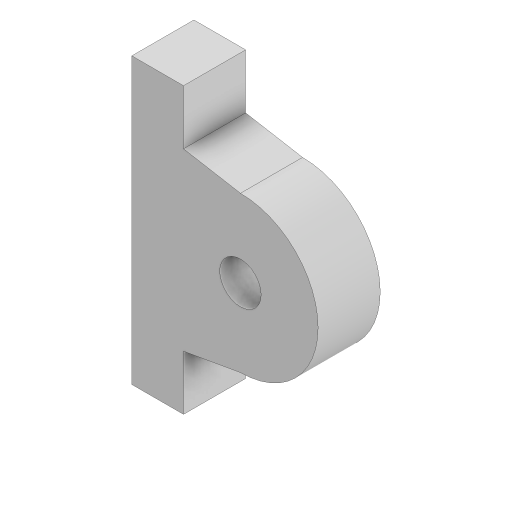
# Autodesk Inventor part: RODAMIENTO DE TORNILLO
Saved by Autodesk Inventor 2024 (Build 280153000, 153)
## iProperties
Created: 2024-06-13
Part Number: RODAMIENTO DE TORNILLO
Material: Generic
Document SubType Name: Modeling
Designer: Jhuliams
Density: 1 g/cm^3
Appearance: Default
Author: Jhuliams
Autodesk Inventor part; units mm, degrees
ref_plane "YZ Plane" through (0, 0, 0) normal (1, 0, 0) x (0, 1, 0)
ref_plane "XZ Plane" through (0, 0, 0) normal (0, 1, 0) x (-1, 0, 0)
ref_plane "XY Plane" through (0, 0, 0) normal (0, 0, 1) x (1, 0, 0)
sketch "Sketch1" plane through (0, 0, 0) normal (0, 0, 1) x (1, 0, 0)
  circle A0 centre (0, 0) radius 4
  circle A1 centre (0, 0) radius 15
  line L0 (0, 16.3344) -> (0, 4)
  line L1 (0, -4) -> (0, -14.3344)
  line L2 (0, 0) -> (-16, 0)
  line L3 (-21, 27.5) -> (-11, 27.5)
  line L4 (-11, 27.5) -> (-11, -27.5)
  line L5 (-11, -27.5) -> (-21, -27.5)
  line L6 (-21, -27.5) -> (-21, 27.5)
  line L7 (-21, 27.5) -> (-11, -27.5) construction
  line L8 (-11, 27.5) -> (-21, -27.5) construction
  line L9 (-16, 27.5) -> (-16, -27.5)
  line L10 (0, -15) -> (-11, -16.9396)
  line L11 (0, -15) -> (11.1697, -15) construction
  line L12 (0, 15) -> (-11, 16.9396)
  point P0 (0, -11)
  point P1 (0, 15)
  point P2 (0, 15)
  dimension "d3" = 30
  dimension "d0" = 8
  dimension "d7" = 16
  dimension "d8" = 10
  dimension "d9" = 55
  dimension "d10" = 170
  constraints: 26 end point, 4 midpoint, 3 horizontal, 2 parallel, 2 point on circle, 2 point on line, 2 symmetric about line, 1 centre point, 1 coincident, 1 equal length, 1 perpendicular, 3 other
  measures "d0" diameter of A0
  measures "d7" distance of L2.start L2.end
  measures "d8" distance of L4.end L5.end
  measures "d9" distance of L3.end L4.end
  measures "d10" angle of L10 L11
extrude "Extrusion1" add sketch "Sketch1" along normal mid plane 12 contours A0 L0 A1 L4 L2 | A0 L2 L4 A1 L0 | A1 L4 L12 | L4 A1 L2 | L2 A1 L4 | A1 L2 L9 L3 L4 | A1 L4 L5 L9 L2 | A1 L10 L4 | L9 L5 L6 L3
body "Solid1"
